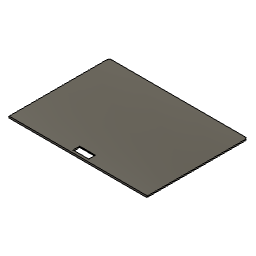
back (Autodesk Fusion 360 design; units mm, degrees)
Autodesk Fusion 360 part; units mm, degrees
sketch "Sketch1" plane through (0, 0, 0) normal (0, 0, 1) x (1, 0, 0)
  line L0 (244.9063, 87.8669) -> (244.9063, -23.3331)
  line L1 (78.2063, -13.5431) -> (78.2063, 84.3769)
  line L2 (241.4063, 84.3769) -> (241.4063, -13.5431)
  line L3 (244.9063, -23.3331) -> (74.7063, -23.3331)
  line L4 (71.3063, 91.2669) -> (248.3063, 91.2669)
  line L5 (244.9063, 87.8669) -> (244.9063, -33.3331)
  line L6 (74.7063, -23.3331) -> (74.7063, 87.8669)
  line L7 (169.8063, -23.3331) -> (149.8063, -23.3331)
  line L8 (169.8063, -33.3331) -> (169.8063, -23.3331)
  line L9 (149.8063, -33.3331) -> (169.8063, -33.3331)
  line L10 (149.8063, -23.3331) -> (149.8063, -33.3331)
  line L11 (74.7063, -33.3331) -> (74.7063, 87.8669)
  line L12 (74.3063, 88.2669) -> (245.3063, 88.2669)
  line L13 (245.3063, 88.2669) -> (245.3063, -23.7331)
  line L14 (74.7063, 87.8669) -> (244.9063, 87.8669)
  line L15 (78.2063, 84.3769) -> (241.4063, 84.3769)
  line L16 (74.7063, 87.8669) -> (244.9063, 87.8669)
  line L17 (74.3063, -23.7331) -> (74.3063, 88.2669)
  line L18 (241.4063, -13.5431) -> (78.2063, -13.5431)
  line L19 (245.3063, -23.7331) -> (74.3063, -23.7331)
  line L20 (248.3063, 91.2669) -> (248.3063, -36.7331)
  line L21 (248.3063, -36.7331) -> (71.3063, -36.7331)
  line L22 (71.3063, -36.7331) -> (71.3063, 91.2669)
  line L23 (244.9063, -33.3331) -> (74.7063, -33.3331)
  line L24 (149.8063, -23.3331) -> (169.8063, -23.3331)
  line L25 (169.8063, -23.3331) -> (169.8063, -25.3329)
  line L26 (169.8063, -25.3329) -> (149.8063, -25.3329)
  line L27 (149.8063, -25.3329) -> (149.8063, -23.3331)
  dimension "d1" = -3.4
  dimension "d2" = -0.4
  dimension "d3" = 97.92
  dimension "d4" = 163.2
  dimension "d5" = 170.2
  dimension "d6" = 3.5
  dimension "d7" = 111.2
  dimension "d8" = 3.49
  dimension "d9" = 10
  dimension "d10" = 20
  dimension "d11" = 75.1
  dimension "d12" = 75.1
  constraint horizontal L15
  constraint vertical L2
  constraint horizontal L18
  constraint vertical L1
  constraint horizontal L16
  constraint vertical L0
  constraint horizontal L3
  constraint vertical L6
  constraint horizontal L14
  constraint vertical L5
  constraint horizontal L23
  constraint vertical L11
  constraint horizontal L9
  constraint vertical L8
  constraint horizontal L7
  constraint vertical L10
  constraint coincident L7.start L3
  constraint coincident L9.start L23
  constraint horizontal L24
  constraint vertical L25
  constraint horizontal L26
  constraint vertical L27
  constraint coincident L8 L25.end
  measures "d3" distance of L1.end L1.start
  measures "d4" distance of L1.end L2.start
  measures "d5" distance of L0.start L6.end
  measures "d6" distance of L1 L6
  measures "d7" distance of L6.end L3.end
  measures "d8" distance of L15 L16
  measures "d9" distance of L3 L23
  measures "d10" distance of L8.start L9.start
  measures "d11" distance of L10 L11
  measures "d12" distance of L5 L8
extrude "Extrude1" add sketch "Sketch1" along normal blind 1.5 contours L0 L5 L6 L11 L12 L13 L14 L16 L17 L19 | L0 L3 L5 L6 L7 L11 L14 L16 L24 | L3 L5 L8 L19 L25 | L3 L7 L8 L10 L19 L24 L25 L27 | L5 L8 L19 L23 L25 | L3 L10 L11 L19 L27 | L8 L10 L19 L25 L26 L27 | L10 L11 L19 L23 L27 | L1 L2 L15 L18 | L4 L20 L21 L22
fillet "Fillet1" radius 3 2 edges at (248.3063, 91.2669, 0.75) (71.3063, 91.2669, 0.75)
fillet "Fillet2" radius 0.5 2 edges at (159.8063, -25.3329, 0) (159.8063, -25.3329, 1.5)
sketch "Sketch2" plane through (248.3063, 0, 0) normal (1, 0, 0) x (0, 1, 0)
  line L0 (88.2669, 0) -> (88.2669, 1.5)
  line L1 (88.2669, 1.5) -> (-36.7331, 1.5)
  line L2 (-36.7331, 1.5) -> (-36.7331, 0)
  line L3 (-36.7331, 0) -> (88.2669, 0)
  line L4 (-36.7331, 1.5) -> (-37.9806, -1.1754)
  line L5 (-36.7331, 1.5) -> (-33.7811, 1.5) construction
  line L6 (-36.7331, 0) -> (-38.6066, 0)
  dimension "d19" = 115
  constraint horizontal L5
  constraint coincident L1.end L2.start
  constraint coincident L2.end L3.start
  constraint perpendicular L2 L6
  measures "d19" angle of L4 L5
extrude "Extrude2" add sketch "Sketch2" against normal up to surface (177 mm away) contours L2 L4 L6
